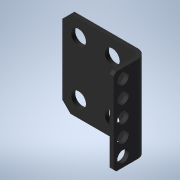
# Autodesk Inventor part: 8617.540_P2
Saved by Autodesk Inventor 2021 (Build 250183000, 183)
## iProperties
Created: 2026-08-04
Part Number: 8617.540_P2
Material: Generic
Catalog Web Link: www.3dfindit.com
Description: VX Teilmontageplatte - P2-VX Teilmontageplatte - P2
Vendor: RITTAL
Document SubType Name: Modeling
Designer: psAdmin
Manufacturer: RITTAL
Mass: 13.1792 g
Surface Area: 104.351 cm^2
Volume: 13.1792 cm^3
Density: 1 g/cm^3
Appearance: PSOLRGB-176-176-176
Category: PARTsolutions
Company: RITTAL
Title: 8617.540_P2
Author: Cadenas PARTsolutions
Comments: VX Teilmontageplatte - P2
PSOL_IDENT_0: {$CADENAS_DATA/23d-libs/rittal/sys_zub/innenausbau/montageplatten/parts/teilmontageplatten_m51_p2.pr
PSOL_IDENT_1: j},181 {VTYP=3D},{NB=8617.540_P2},{LINA=8617.540_P2},{NN=VX Teilmontageplatte - P2},{DATE=16.02.2026
PSOL_IDENT_2: 20:13:30},{GEOMDATE=11.04.2025 11:24:24},{VERSION=},{LINEID=40},{WBVAR=},{WBNUMERIC=}  {NB=8617.540
PSOL_IDENT_3: _P2},{LINA=8617.540_P2},{KT=DUMMY},{BEST=8617.540},{INFO=PDF Katalog},{BEZ1=VX Teilmontageplatte},{B
PSOL_IDENT_4: EZ2=für neues Großschranksystem},{B=600},{BB=499},{H=800},{HH=699},{SB=600},{SH=800},{AB=600 x 800},
PSOL_IDENT_5: {VE=1},{VERS=4},{INFOPAGE=hb35_s707},{INFOPATH=hb35_s707_en.pdf},{CNSECLASS51=27-18-92-31},{CNSECLAS
PSOL_IDENT_6: S70=27-40-92-16},{CNSECLASS80=27-40-92-16},{CNSETIM40=EC000213},{BEZ3=},{DETAIL=1},{ADDGEO=1},{GEW=9
PSOL_IDENT_7: ,22},{CNSETIM80=EC000213},{CNSETIM90=EC000213},{CNSECLASS60=27-40-92-16},{UNSPSC=31-26-15-02}
NB: 8617.540_P2
NN: VX Teilmontageplatte - P2
NT: VX Teilmontageplatte - P2
NBSYN: $BEST._P2
LINA: 8617.540_P2
CATALOG: Rittal
BEST: 8617.540
INFO: PDF Katalog
BEZ1: VX Teilmontageplatte
BB: 499
HH: 699
SB: 600
SH: 800
CNSECLASS70: 27-40-92-16
CNSECLASS80: 27-40-92-16
GEW: 9,22
CNSETIM80: EC000213
CNSETIM90: EC000213
CNSECLASS60: 27-40-92-16
UNSPSC: 31-26-15-02
SUPPLIER: RITTAL
ARTICLENO: 8617.540_P2
BOMINFO: 8617.540_P2
CREATOR: CADENAS GmbH
Autodesk Inventor part; units mm, degrees
sketch "Sketch_8" plane through (0, 0, 0) normal (0, 0, 1) x (1, 0, 0)
  line L0 (-37, 26) -> (-37, -26)
  line L1 (-37, -26) -> (-31, -32)
  line L2 (-31, -32) -> (16, -32)
  line L3 (16, -32) -> (16, 32)
  line L4 (16, 32) -> (-31, 32)
  line L5 (-31, 32) -> (-37, 26)
  circle A0 centre (0, -20) radius 5.5
  circle A1 centre (0, 20) radius 5.5
  circle A2 centre (-25, -20) radius 5.5
  circle A3 centre (-25, 20) radius 5.5
  constraints: 12 end point, 4 centre point
extrude "Extrusion1" add sketch "Sketch_8" against normal blind 3
sketch "Sketch_1" plane through (0, 0, 0) normal (0, 1, 0) x (1, 0, 0)
  arc A0 (20, -4) -> (16, 0) centre (16, -4) ccw
  line L0 (20, -4) -> (23, -4)
  arc A1 (23, -4) -> (16, 3) centre (16, -4) ccw
  line L1 (16, 3) -> (16, 0)
  constraints: 4 end point, 4 point on circle, 2 centre point
extrude "Extrusion2" add sketch "Sketch_1" along normal mid plane 64
sketch "Sketch_2" plane through (23, 0, 0) normal (1, 0, 0) x (0, 0, -1)
  line L0 (-22, -30) -> (-20, -32)
  line L1 (-20, -32) -> (-4, -32)
  line L2 (-4, -32) -> (-4, 32)
  line L3 (-4, 32) -> (-20, 32)
  line L4 (-20, 32) -> (-22, 30)
  line L5 (-22, 30) -> (-22, -30)
  circle A0 centre (-15, -25) radius 4.25
  circle A1 centre (-15, -12.5) radius 4.25
  circle A2 centre (-15, 0) radius 4.25
  circle A3 centre (-15, 12.5) radius 4.25
  circle A4 centre (-15, 25) radius 4.25
  constraints: 12 end point, 5 centre point
extrude "Extrusion3" add sketch "Sketch_2" against normal blind 3
ref_plane "P21_XY" through (0, 20, 0) normal (0, 0, -1) x (1, 0, 0)
ref_plane "P21_YZ" through (0, 20, 0) normal (1, 0, 0) x (0, -1, 0)
ref_plane "P21_ZX" through (0, 20, 0) normal (0, -1, 0) x (0, 0, -1)
ref_plane "P22_XY" through (0, -20, 0) normal (0, 0, -1) x (1, 0, 0)
ref_plane "P22_YZ" through (0, -20, 0) normal (1, 0, 0) x (0, -1, 0)
ref_plane "P22_ZX" through (0, -20, 0) normal (0, -1, 0) x (0, 0, -1)
body "Solid1"
